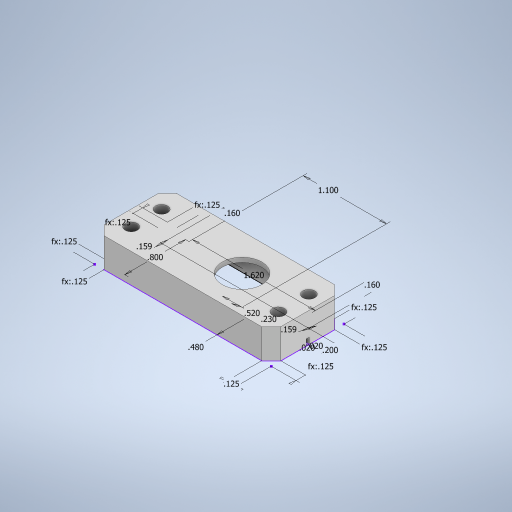
# Autodesk Inventor part: Servo Test Mount
Saved by Autodesk Inventor 2023 (Build 270158000, 158)
## iProperties
Created: 2023-03-13
Part Number: Servo Test Mount
Material: Generic
Document SubType Name: Modeling
Designer: tommy
Density: 1 g/cm^3
Appearance: Default
Author: tommy
Autodesk Inventor part; units mm, degrees
ref_plane "YZ Plane" through (0, 0, 0) normal (1, 0, 0) x (0, 1, 0)
ref_plane "XZ Plane" through (0, 0, 0) normal (0, 1, 0) x (-1, 0, 0)
ref_plane "XY Plane" through (0, 0, 0) normal (0, 0, 1) x (1, 0, 0)
sketch "Sketch1" plane through (0, 0, 0) normal (0, 1, 0) x (-1, 0, 0)
  line L0 (0, 0) -> (41.148, 0)
  line L1 (41.148, 0) -> (41.148, -20.32)
  line L2 (41.148, -20.32) -> (0, -20.32)
  line L3 (0, -20.32) -> (0, 0)
  line L4 (47.498, 2.0259) -> (-5.588, 2.0259)
  line L5 (-5.588, -22.3459) -> (47.1979, -22.3459)
  circle A0 centre (45.212, -15.24) radius 2.0193
  circle A1 centre (-4.064, -15.24) radius 2.0193
  line L6 (-8.7354, -10.16) -> (50.3729, -10.16)
  line L7 (-5.588, 2.0259) -> (-5.5604, 2.0259)
  line L8 (-8.7354, -1.1491) -> (-8.7354, -19.1709)
  line L9 (-5.5604, -22.3459) -> (-5.588, -22.3459)
  line L10 (47.498, -22.3459) -> (47.1979, -22.3459)
  line L11 (50.3729, -19.1709) -> (50.3729, -1.1491)
  line L12 (47.1979, 2.0259) -> (47.498, 2.0259)
  circle A2 centre (45.212, -5.08) radius 2.0193
  circle A3 centre (-4.064, -5.08) radius 2.0193
  line L13 (-5.5604, 2.0259) -> (-8.7354, -1.1491)
  line L14 (-8.7354, -19.1709) -> (-5.5604, -22.3459)
  line L15 (47.1979, -22.3459) -> (50.3729, -19.1709)
  line L16 (50.3729, -1.1491) -> (47.1979, 2.0259)
  circle A4 centre (13.208, -10.16) radius 2.921
  line L17 (-8.7354, -10.668) -> (50.3729, -10.668)
  line L18 (-8.7354, -9.652) -> (50.3729, -9.652)
  circle A5 centre (13.208, -10.16) radius 6.604
  point P0 (-8.7354, 2.0259)
  point P1 (-8.7354, -22.3459)
  point P2 (50.3729, -22.3459)
  point P3 (50.3729, 2.0259)
  point P4 (0, -10.668)
  point P5 (0, -9.652)
  point P6 (41.148, -9.652)
  point P7 (41.148, -10.668)
  dimension "d0" = 41.148
  dimension "d1" = 20.32
  dimension "d4" = 4.0386
  dimension "d5" = 4.0386
  dimension "d16" = 5.08
  dimension "d18" = 4.064
  dimension "d19" = 4.064
  dimension "d20" = 3.175
  dimension "d21" = 3.175
  dimension "d22" = 3.175
  dimension "d23" = 3.175
  dimension "d24" = 3.175
  dimension "d25" = 3.175
  dimension "d26" = 3.175
  dimension "d27" = 3.175
  dimension "d30" = 5.842
  dimension "d31" = 27.94
  dimension "d34" = 0.508
  dimension "d35" = 12.1859
  dimension "d36" = 0.508
  dimension "d39" = 13.208
  constraints: 38 end point, 15 point on line, 7 perpendicular, 6 centre point, 3 parallel, 2 horizontal, 2 midpoint, 1 coincident
  measures "d0" distance of L1.end L2.end
  measures "d1" distance of L0.end L1.end
  measures "d4" diameter of A0
  measures "d5" diameter of A1
  measures "d16" distance from line of L6 A0.centre
  measures "d18" distance from line of L1 A0.centre
  measures "d19" distance from line of L3 A1.centre
  measures "d20" distance of L7.end point (-8.735, 2.026)
  measures "d21" distance of L8.start point (-8.735, 2.026)
  measures "d22" distance of L8.end point (-8.735, -22.346)
  measures "d23" distance of L9.start point (-8.735, -22.346)
  measures "d24" distance of L5.end point (50.373, -22.346)
  measures "d25" distance of L11.start point (50.373, -22.346)
  measures "d26" distance of L11.end point (50.373, 2.026)
  measures "d27" distance of L12.start point (50.373, 2.026)
  measures "d30" diameter of A4
  measures "d31" distance from line of L1 A4.centre
  measures "d34" distance between parallel lines of L6 L17
  measures "d35" distance between parallel lines of L4 L6
  measures "d36" distance between parallel lines of L6 L18
  measures "d39" diameter of A5
extrude "Extrusion7" add sketch "Sketch1" along normal blind 9.8552 contours L3 L18 L8 L13 L4 L16 L11 L1 L0 | L0 L1 L18 A5 L3 | L18 A5 L6 L3 | L3 L6 L8 L18 | L18 L11 L6 L1 | L1 L6 A5 L18 | L6 A5 L17 L3 | L3 L17 L8 L6 | L6 L11 L17 L1 | L1 L17 A5 L6 | L17 A5 L1 L2 L3 | L3 L2 L1 L17 L11 L15 L5 L14 L8
extrude "Extrusion8" cut sketch "Sketch1" along normal blind 8.3312 contours L0 L1 L18 A5 L3 | L18 A5 L6 L3 | L1 L6 A5 L18 | L6 A5 L17 L3 | A5 L18 A4 | L18 A4 L6 A5 | L1 L17 A5 L6 | A5 L6 A4 L18 | L17 A5 L1 L2 L3 | L6 A4 L17 A5 | L18 A4 L6 | A4 L18 | A5 L17 A4 L6 | L17 A4 A5 | L6 A4 L17 | L17 A4
extrude "Extrusion9" cut sketch "Sketch1" along normal blind 2.032 contours L3 L6 L8 L18 | L18 L11 L6 L1 | L3 L17 L8 L6 | L6 L11 L17 L1
equation "\"d21\" = d20"
equation "\"d22\" = d20"
equation "\"d23\" = d22"
equation "\"d24\" = d20"
equation "\"d25\" = d24"
equation "\"d26\" = d20"
equation "\"d27\" = d26"
body "Solid3"
